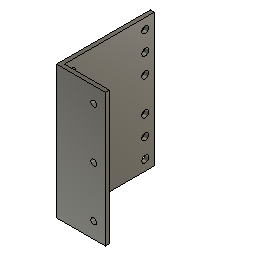
Front MotorController Holder v1 (Autodesk Fusion 360 design; units mm, degrees)
Autodesk Fusion 360 part; units mm, degrees
sketch "Sketch1" plane through (0, 0, 0) normal (0, 0, 1) x (1, 0, 0)
  line L0 (0, 0) -> (-25, 0)
  line L1 (-25, 0) -> (-25, 48)
  line L2 (-25, 48) -> (-23, 48)
  line L3 (-23, 48) -> (-23, 2)
  line L4 (-23, 2) -> (0, 2)
  line L5 (0, 2) -> (0, 0)
  dimension "d1" = 2
  dimension "d2" = 23
  dimension "d3" = 25
  dimension "d35" = 2
  constraint coincident L0.start L5.end
  constraint horizontal L0
  constraint perpendicular L0 L1
  constraint perpendicular L1 L2
  constraint perpendicular L2 L3
  constraint perpendicular L3 L4
  measures "d1" distance of L1.end L2.end
  measures "d2" distance of L3.end L4.end
  measures "d3" distance of L0.start L0.end
  measures "d35" distance of L4.end L0.start
extrude "Extrude1" add sketch "Sketch1" along normal blind 68
sketch "Sketch2" plane through (-25, 0, 0) normal (-1, 0, 0) x (0, -1, 0)
  line L0 (-48, 0) -> (0, 0)
  line L1 (0, 0) -> (0, 68)
  line L2 (0, 68) -> (-48, 68)
  line L3 (-48, 68) -> (-48, 0)
  circle A0 centre (-6, 52.65) radius 1.75
  dimension "d8" = 3.5
  dimension "d9" = 15.35
  dimension "d10" = 6
  measures "d8" diameter of A0
  measures "d9" distance of L2 A0.centre
  measures "d10" distance of L1 A0.centre
extrude "Extrude2" cut sketch "Sketch2" against normal blind 15 contours A0
pattern_linear "R-Pattern1" count 1 spacing 0 along (0, 1, 0) count 2 spacing 37.3 along (0, 0, -1) of "Extrude2"
sketch "Sketch3" plane through (-25, 0, 0) normal (-1, 0, 0) x (0, -1, 0)
  circle A0 centre (-6, 15.35) radius 1.75
  circle A1 centre (-6, 52.65) radius 1.75
  line L0 (-48, 0) -> (0, 0)
  line L1 (0, 0) -> (0, 68)
  line L2 (0, 68) -> (-48, 68)
  line L3 (-48, 68) -> (-48, 0)
  circle A2 centre (-43.3, 52.65) radius 1.75
  dimension "d17" = 3.5
  dimension "d18" = 15.35
  dimension "d19" = 37.3
  measures "d17" diameter of A2
  measures "d18" distance of L2 A2.centre
  measures "d19" distance of A1.centre A2.centre
extrude "Extrude3" cut sketch "Sketch3" against normal blind 10 contours A2
pattern_linear "R-Pattern2" count 2 spacing 37.3 along (0, 0, -1) of "Extrude3"
sketch "Sketch4" plane through (0, 0, 0) normal (0, -1, 0) x (1, 0, 0)
  line L0 (-25, 0) -> (0, 0)
  line L1 (0, 0) -> (0, 68)
  line L2 (0, 68) -> (-25, 68)
  line L3 (-25, 68) -> (-25, 0)
  circle A0 centre (-6, 60) radius 1.475
  dimension "d26" = 2.95
  dimension "d27" = 8
  dimension "d28" = 6
  measures "d26" diameter of A0
  measures "d27" distance of L2 A0.centre
  measures "d28" distance of L1 A0.centre
extrude "Extrude4" cut sketch "Sketch4" against normal blind 6 contours A0
pattern_linear "R-Pattern3" count 3 spacing 26 along (0, 0, -1) of "Extrude4"
pattern_linear "R-Pattern4" count 2 spacing 10 along (0, 0, 1) of "Extrude2", "R-Pattern1", "Extrude3", "R-Pattern2"
pattern_linear "R-Pattern5" count 2 spacing 10 along (0, 0, -1) of "Extrude2", "R-Pattern1", "Extrude3", "R-Pattern2"
